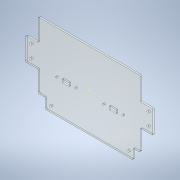
# Autodesk Inventor part: BackAcrylicSheet
Saved by Autodesk Inventor 2021 (Build 250183000, 183)
## iProperties
Created: 2020-07-16
Part Number: BackAcrylicSheet
Material: Generic
Document SubType Name: Modeling
Designer: CASE-SMALL2
Density: 1 g/cm^3
Appearance: Default
Author: CASE-SMALL2
Autodesk Inventor part; units mm, degrees
ref_plane "YZ Plane" through (0, 0, 0) normal (1, 0, 0) x (0, 1, 0)
ref_plane "XZ Plane" through (0, 0, 0) normal (0, 1, 0) x (-1, 0, 0)
ref_plane "XY Plane" through (0, 0, 0) normal (0, 0, 1) x (1, 0, 0)
sketch "Sketch1" plane through (0, 0, 0) normal (0, 0, 1) x (1, 0, 0)
  line L0 (-125, -75) -> (125, -75)
  line L1 (125, -75) -> (125, 75)
  line L2 (125, 75) -> (-125, 75)
  line L3 (-125, 75) -> (-125, -75)
  line L4 (-125, -75) -> (125, 75) construction
  line L5 (125, -75) -> (-125, 75) construction
  point P0 (0, 0)
  dimension "d0" = 150
  dimension "d1" = 250
  constraints: 12 end point, 2 midpoint, 2 parallel, 1 horizontal, 1 perpendicular
  measures "d0" distance of L2.end L0.start
  measures "d1" distance of L1.end L2.end
extrude "Extrusion1" add sketch "Sketch1" along normal blind 3
sketch "Sketch2" plane through (0, 0, 3) normal (0, 0, 1) x (1, 0, 0)
  line L0 (125, -75) -> (125, 75) construction
  line L1 (125, 75) -> (-125, 75) construction
  line L2 (-125, 75) -> (-125, -75) construction
  line L3 (-125, -75) -> (125, -75) construction
  line L4 (-125, 75) -> (-125, -75) construction
  line L5 (125, 75) -> (-125, 75) construction
  line L6 (-125, 75) -> (-100, 75)
  line L7 (-100, 75) -> (-100, 31)
  line L8 (-100, 31) -> (-125, 31)
  line L9 (-125, 31) -> (-125, 75)
  line L10 (-125, -14) -> (-100, -14)
  line L11 (-100, -14) -> (-100, -55)
  line L12 (-100, -55) -> (-86, -55)
  line L13 (-86, -55) -> (-86, -75)
  line L14 (-125, -75) -> (125, -75) construction
  line L15 (-125, -14) -> (-125, -75)
  line L16 (-125, -75) -> (-86, -75)
  line L17 (0, -105) -> (0, 105) construction
  line L18 (125, 75) -> (125, -75) construction
  line L19 (125, 75) -> (125, -75) construction
  line L20 (125, 75) -> (100, 75)
  line L21 (100, 75) -> (100, 31)
  line L22 (100, 31) -> (125, 31)
  line L23 (125, 31) -> (125, 75)
  line L24 (125, -14) -> (100, -14)
  line L25 (100, -14) -> (100, -55)
  line L26 (100, -55) -> (86, -55)
  line L27 (86, -55) -> (86, -75)
  line L28 (125, -14) -> (125, -75)
  line L29 (125, -75) -> (86, -75)
  point P0 (0, 0)
  dimension "d4" = 25
  dimension "d5" = 44
  dimension "d6" = 25
  dimension "d7" = 20
  dimension "d10" = 39
  dimension "d11" = 61
  constraints: 44 end point, 8 symmetric about line, 3 perpendicular, 3 point on line, 2 collinear, 2 horizontal, 2 parallel, 1 vertical
  measures "d4" distance between parallel lines of L2 L7
  measures "d5" distance between parallel lines of L1 L8
  measures "d6" distance between parallel lines of L2 L11
  measures "d7" distance between parallel lines of L3 L12
  measures "d10" distance between parallel lines of L4 L13
  measures "d11" distance between parallel lines of L10 L16
extrude "Extrusion2" cut sketch "Sketch2" against normal blind 3
sketch "Sketch3" plane through (0, 0, 3) normal (0, 0, 1) x (1, 0, 0)
  point P0 (0, 0)
fillet "Fillet1" radius 2 15 edges at (86, -75, 1.5) (86, -55, 1.5) (100, -55, 1.5) (100, -14, 1.5) (125, -14, 1.5) (125, 31, 1.5) (100, 75, 1.5) (-100, 75, 1.5) (-100, 31, 1.5) (-125, 31, 1.5) (-125, -14, 1.5) (-100, -14, 1.5) (-100, -55, 1.5) (-86, -55, 1.5) (-86, -75, 1.5)
sketch "Sketch4" plane through (0, 0, 3) normal (0, 0, 1) x (1, 0, 0)
  circle A0 centre (-115, 21) radius 2.25
  circle A1 centre (-115, -4) radius 2.25
  circle A2 centre (-76, -65) radius 2.25
  line L0 (-125, 29) -> (-125, -12) construction
  line L1 (-102, 31) -> (-123, 31) construction
  line L2 (-123, -14) -> (-102, -14) construction
  line L3 (-86, -57) -> (-86, -73) construction
  line L4 (-84, -75) -> (84, -75) construction
  line L5 (0, -105) -> (0, 105) projected
  circle A3 centre (115, 21) radius 2.25
  circle A4 centre (115, -4) radius 2.25
  circle A5 centre (76, -65) radius 2.25
  line L6 (125, 29) -> (125, -12) construction
  line L7 (102, 31) -> (123, 31) construction
  line L8 (123, -14) -> (102, -14) construction
  line L9 (86, -57) -> (86, -73) construction
  point P0 (0, 0)
  dimension "d13" = 4.5
  dimension "d14" = 4.5
  dimension "d15" = 4.5
  dimension "d16" = 10
  dimension "d17" = 10
  dimension "d18" = 10
  dimension "d19" = 10
  dimension "d20" = 10
  dimension "d21" = 10
  constraints: 11 symmetric about line, 8 end point, 6 centre point, 3 other
  measures "d13" diameter of A0
  measures "d14" diameter of A1
  measures "d15" diameter of A2
  measures "d16" distance from line of L0 A0.centre
  measures "d17" distance from line of L1 A0.centre
  measures "d18" distance from line of L0 A1.centre
  measures "d19" distance from line of L2 A1.centre
  measures "d20" distance from line of L3 A2.centre
  measures "d21" distance from line of L4 A2.centre
extrude "Extrusion3" cut sketch "Sketch4" against normal blind 3
sketch "Sketch6" plane through (0, 0, 3) normal (0, 0, 1) x (1, 0, 0)
  circle A0 centre (65, -10) radius 1.75
  line L0 (65, -10) -> (27.4, -10) construction
  circle A1 centre (27.4, -10) radius 1.75
  line L1 (-84, -75) -> (84, -75) projected
  line L2 (100, -53) -> (100, -16) projected
  line L3 (0, -105.5799) -> (0, 105.5799) projected
  circle A2 centre (-65, -10) radius 1.75
  line L4 (-65, -10) -> (-27.4, -10) construction
  circle A3 centre (-27.4, -10) radius 1.75
  line L5 (27.4, -10) -> (65, -10) construction
  line L6 (39.4, -13.1) -> (53, -13.1)
  line L7 (53, -13.1) -> (53, -6.9)
  line L8 (53, -6.9) -> (39.4, -6.9)
  line L9 (39.4, -6.9) -> (39.4, -13.1)
  line L10 (39.4, -13.1) -> (53, -6.9) construction
  line L11 (53, -13.1) -> (39.4, -6.9) construction
  line L12 (-39.4, -13.1) -> (-53, -13.1)
  line L13 (-53, -13.1) -> (-53, -6.9)
  line L14 (-53, -6.9) -> (-39.4, -6.9)
  line L15 (-39.4, -6.9) -> (-39.4, -13.1)
  line L16 (-39.4, -13.1) -> (-53, -6.9) construction
  line L17 (-53, -13.1) -> (-39.4, -6.9) construction
  point P0 (0, 0)
  point P1 (46.2, -10)
  point P2 (-46.2, -10)
  dimension "d24" = 3.5
  dimension "d25" = 3.5
  dimension "d26" = 37.6
  dimension "d27" = 65
  dimension "d28" = 35
  dimension "d31" = 13.6
  dimension "d32" = 6.2
  dimension "d33" = 18.8
  dimension "d34" = 18.8
  constraints: 30 end point, 8 symmetric about line, 5 midpoint, 4 centre point, 3 horizontal, 2 coincident, 2 parallel, 1 perpendicular, 2 other
  measures "d24" diameter of A0
  measures "d25" diameter of A1
  measures "d26" distance of L0.start L0.end
  measures "d27" distance from line of L1 L0.end
  measures "d28" distance from line of L2 L0.start
  measures "d31" distance of L7.end L8.end
  measures "d32" distance of L6.end L7.end
  measures "d33" distance of L0.start point (46.2, -10)
  measures "d34" distance of L0.end point (46.2, -10)
extrude "Extrusion4" cut sketch "Sketch6" against normal blind 10
sketch "Sketch8" plane through (0, 0, 3) normal (0, 0, 1) x (1, 0, 0)
  circle A0 centre (-65, -10) radius 1.75 projected
  circle A1 centre (65, -10) radius 1.75 projected
  line L0 (39.4, -6.9) -> (53, -6.9) projected
  line L1 (53, -6.9) -> (53, -13.1) projected
  line L2 (53, -13.1) -> (39.4, -13.1) projected
  line L3 (39.4, -13.1) -> (39.4, -6.9) projected
  circle A2 centre (-27.4, -10) radius 1.75 projected
  circle A3 centre (27.4, -10) radius 1.75 projected
  line L4 (-39.4, -13.1) -> (-53, -13.1) projected
  line L5 (-53, -13.1) -> (-53, -6.9) projected
  line L6 (-53, -6.9) -> (-39.4, -6.9) projected
  line L7 (-39.4, -6.9) -> (-39.4, -13.1) projected
  circle A4 centre (-76, -65) radius 2.25 projected
  circle A5 centre (115, 21) radius 2.25 projected
  circle A6 centre (-115, -4) radius 2.25 projected
  circle A7 centre (76, -65) radius 2.25 projected
  circle A8 centre (115, -4) radius 2.25 projected
  circle A9 centre (-115, 21) radius 2.25 projected
  arc A10 (-86, -73) -> (-84, -75) centre (-84, -73) ccw projected
  line L8 (-84, -75) -> (84, -75) projected
  arc A11 (84, -75) -> (86, -73) centre (84, -73) ccw projected
  line L9 (86, -73) -> (86, -57) projected
  arc A12 (88, -55) -> (86, -57) centre (88, -57) ccw projected
  line L10 (88, -55) -> (98, -55) projected
  arc A13 (98, -55) -> (100, -53) centre (98, -53) ccw projected
  line L11 (100, -53) -> (100, -16) projected
  arc A14 (102, -14) -> (100, -16) centre (102, -16) ccw projected
  line L12 (102, -14) -> (123, -14) projected
  arc A15 (123, -14) -> (125, -12) centre (123, -12) ccw projected
  line L13 (125, -12) -> (125, 29) projected
  arc A16 (125, 29) -> (123, 31) centre (123, 29) ccw projected
  line L14 (123, 31) -> (100, 31) projected
  line L15 (100, 31) -> (100, 73) projected
  arc A17 (100, 73) -> (98, 75) centre (98, 73) ccw projected
  line L16 (98, 75) -> (-98, 75) projected
  arc A18 (-98, 75) -> (-100, 73) centre (-98, 73) ccw projected
  line L17 (-100, 73) -> (-100, 33) projected
  arc A19 (-102, 31) -> (-100, 33) centre (-102, 33) ccw projected
  line L18 (-102, 31) -> (-123, 31) projected
  arc A20 (-123, 31) -> (-125, 29) centre (-123, 29) ccw projected
  line L19 (-125, 29) -> (-125, -12) projected
  arc A21 (-125, -12) -> (-123, -14) centre (-123, -12) ccw projected
  line L20 (-123, -14) -> (-102, -14) projected
  arc A22 (-100, -16) -> (-102, -14) centre (-102, -16) ccw projected
  line L21 (-100, -16) -> (-100, -53) projected
  arc A23 (-100, -53) -> (-98, -55) centre (-98, -53) ccw projected
  line L22 (-98, -55) -> (-88, -55) projected
  arc A24 (-86, -57) -> (-88, -55) centre (-88, -57) ccw projected
  line L23 (-86, -57) -> (-86, -73) projected
  point P0 (0, 0)
equation "\"d6\" = d4"
equation "\"d14\" = d13"
equation "\"d15\" = d14"
equation "\"d17\" = d16"
equation "\"d18\" = d16"
equation "\"d19\" = d16"
equation "\"d20\" = d19"
equation "\"d21\" = d19"
equation "\"d25\" = d24"
body "Solid1"
